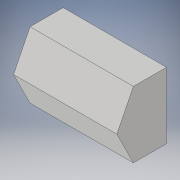
# Autodesk Inventor part: UWO-BLWT-SS21-Test6-40ft
Saved by Autodesk Inventor 2017 (Build 210142000, 142)
## iProperties
Created: 2018-11-14
Part Number: UWO-BLWT-SS21-Test6-40ft
Material: Generic
Document SubType Name: Modeling
Designer: mcgratta
Density: 1 g/cm^3
Appearance: Default
Author: mcgratta
Autodesk Inventor part; units mm, degrees
ref_plane "YZ Plane" through (0, 0, 0) normal (1, 0, 0) x (0, 1, 0)
ref_plane "XZ Plane" through (0, 0, 0) normal (0, 1, 0) x (-1, 0, 0)
ref_plane "XY Plane" through (0, 0, 0) normal (0, 0, 1) x (1, 0, 0)
sketch "Sketch1" plane through (0, 0, 0) normal (1, 0, 0) x (0, 1, 0)
  line L0 (0, 0) -> (0, 122)
  line L1 (0, 122) -> (-122, 183)
  line L2 (-122, 183) -> (-244, 122)
  line L3 (-244, 122) -> (-244, 0)
  line L4 (-244, 0) -> (0, 0)
  dimension "d0" = 122
  dimension "d1" = 244
  dimension "d2" = 122
  dimension "d3" = 183
  dimension "d4" = 122
  constraints: 10 end point, 1 parallel, 1 perpendicular, 1 vertical
  measures "d0" distance of L0.start L0.end
  measures "d1" distance of L3.end L0.start
  measures "d2" distance of L2.end L3.end
  measures "d3" distance from line of L4 L1.end
  measures "d4" distance from line of L0 L1.end
extrude "Extrusion1" add sketch "Sketch1" along normal blind 381
body "Solid1"
